Autodesk Inventor part; units mm, degrees
(part 2 of 3)
  line L186 (-35.1562, 49.0328) -> (-35.1562, 44.7064)
  spline S339 degree 2 poles (-35.1562, 44.7064) (-35.1562, 44.3627) (-35.4862, 44.3627) knots 0 0 0 1 1 1
  spline S340 degree 2 poles (-35.4862, 44.3627) (-35.7062, 44.3627) (-35.8666, 44.601) knots 0 0 0 1 1 1
  line L187 (-35.8666, 44.601) -> (-38.1443, 48.1025)
  line L188 (-38.1443, 48.1025) -> (-38.1443, 44.7248)
  spline S341 degree 2 poles (-38.1443, 44.7248) (-38.1443, 44.3627) (-38.4926, 44.3627) knots 0 0 0 1 1 1
  spline S342 degree 2 poles (-38.4926, 44.3627) (-38.8409, 44.3627) (-38.8409, 44.7248) knots 0 0 0 1 1 1
  line L189 (-38.8409, 44.7248) -> (-38.8409, 49.042)
  spline S343 degree 2 poles (-43.4515, 49.042) (-43.4515, 49.3949) (-43.1444, 49.3949) knots 0 0 0 1 1 1
  spline S344 degree 2 poles (-43.1444, 49.3949) (-42.9428, 49.3949) (-42.8098, 49.2024) knots 0 0 0 1 1 1
  line L190 (-42.8098, 49.2024) -> (-40.4633, 45.6093)
  line L191 (-40.4633, 45.6093) -> (-40.4633, 49.0328)
  spline S345 degree 2 poles (-40.4633, 49.0328) (-40.4633, 49.3949) (-40.115, 49.3949) knots 0 0 0 1 1 1
  spline S346 degree 2 poles (-40.115, 49.3949) (-39.7667, 49.3949) (-39.7667, 49.0328) knots 0 0 0 1 1 1
  line L192 (-39.7667, 49.0328) -> (-39.7667, 44.7064)
  spline S347 degree 2 poles (-39.7667, 44.7064) (-39.7667, 44.3627) (-40.0967, 44.3627) knots 0 0 0 1 1 1
  spline S348 degree 2 poles (-40.0967, 44.3627) (-40.3167, 44.3627) (-40.4771, 44.601) knots 0 0 0 1 1 1
  line L193 (-40.4771, 44.601) -> (-42.7548, 48.1025)
  line L194 (-42.7548, 48.1025) -> (-42.7548, 44.7248)
  spline S349 degree 2 poles (-42.7548, 44.7248) (-42.7548, 44.3627) (-43.1032, 44.3627) knots 0 0 0 1 1 1
  spline S350 degree 2 poles (-43.1032, 44.3627) (-43.4515, 44.3627) (-43.4515, 44.7248) knots 0 0 0 1 1 1
  line L195 (-43.4515, 44.7248) -> (-43.4515, 49.042)
  spline S351 degree 2 poles (-56.2885, 49.042) (-56.2885, 49.404) (-55.9402, 49.404) knots 0 0 0 1 1 1
  spline S352 degree 2 poles (-55.9402, 49.404) (-55.5873, 49.404) (-55.5873, 49.042) knots 0 0 0 1 1 1
  line L196 (-55.5873, 49.042) -> (-55.5873, 44.436)
  line L197 (-55.5873, 44.436) -> (-54.1986, 46.6313)
  spline S353 degree 2 poles (-54.1986, 46.6313) (-54.0382, 46.865) (-53.8091, 46.865) knots 0 0 0 1 1 1
  spline S354 degree 2 poles (-53.8091, 46.865) (-53.5891, 46.865) (-53.4745, 46.6955) knots 0 0 0 1 1 1
  line L198 (-53.4745, 46.6955) -> (-52.0584, 44.4177)
  line L199 (-52.0584, 44.4177) -> (-52.0584, 49.042)
  spline S355 degree 2 poles (-52.0584, 49.042) (-52.0584, 49.404) (-51.7009, 49.404) knots 0 0 0 1 1 1
  spline S356 degree 2 poles (-51.7009, 49.404) (-51.348, 49.404) (-51.348, 49.042) knots 0 0 0 1 1 1
  line L200 (-51.348, 49.042) -> (-51.348, 43.7211)
  spline S357 degree 2 poles (-51.348, 43.7211) (-51.348, 43.3407) (-51.7284, 43.3407) knots 0 0 0 1 1 1
  spline S358 degree 2 poles (-51.7284, 43.3407) (-52.0217, 43.3407) (-52.2142, 43.6111) knots 0 0 0 1 1 1
  line L201 (-52.2142, 43.6111) -> (-53.8183, 45.9805)
  line L202 (-53.8183, 45.9805) -> (-55.459, 43.5836)
  spline S359 degree 2 poles (-55.459, 43.5836) (-55.6469, 43.304) (-55.9127, 43.304) knots 0 0 0 1 1 1
  spline S360 degree 2 poles (-55.9127, 43.304) (-56.2885, 43.304) (-56.2885, 43.7165) knots 0 0 0 1 1 1
  line L203 (-56.2885, 43.7165) -> (-56.2885, 49.042)
  spline S361 degree 2 poles (-61.2748, 46.8925) (-61.2748, 47.8641) (-60.7844, 48.5928) knots 0 0 0 1 1 1
  spline S362 degree 2 poles (-60.7844, 48.5928) (-60.2437, 49.3949) (-59.3958, 49.3949) knots 0 0 0 1 1 1
  spline S363 degree 2 poles (-59.3958, 49.3949) (-58.5479, 49.3949) (-58.0071, 48.5837) knots 0 0 0 1 1 1
  spline S364 degree 2 poles (-58.0071, 48.5837) (-57.5213, 47.855) (-57.5213, 46.8925) knots 0 0 0 1 1 1
  spline S365 degree 2 poles (-57.5213, 46.8925) (-57.5213, 45.9347) (-58.0026, 45.2243) knots 0 0 0 1 1 1
  spline S366 degree 2 poles (-58.0026, 45.2243) (-58.5663, 44.404) (-59.3958, 44.404) knots 0 0 0 1 1 1
  spline S367 degree 2 poles (-59.3958, 44.404) (-60.2803, 44.404) (-60.7524, 45.1693) knots 0 0 0 1 1 1
  spline S368 degree 2 poles (-60.7524, 45.1693) (-61.2748, 45.9209) (-61.2748, 46.8925) knots 0 0 0 1 1 1
  spline S369 degree 2 poles (-60.5782, 46.8925) (-60.5782, 46.1776) (-60.3124, 45.7193) knots 0 0 0 1 1 1
  spline S370 degree 2 poles (-60.3124, 45.7193) (-59.9687, 45.1098) (-59.3958, 45.1098) knots 0 0 0 1 1 1
  spline S371 degree 2 poles (-59.3958, 45.1098) (-58.8596, 45.1098) (-58.5204, 45.678) knots 0 0 0 1 1 1
  spline S372 degree 2 poles (-58.5204, 45.678) (-58.218, 46.1913) (-58.218, 46.8925) knots 0 0 0 1 1 1
  spline S373 degree 2 poles (-58.218, 46.8925) (-58.218, 47.6121) (-58.3738, 48.0795) knots 0 0 0 1 1 1
  spline S374 degree 2 poles (-58.3738, 48.0795) (-58.8412, 48.6891) (-59.3958, 48.6891) knots 0 0 0 1 1 1
  spline S375 degree 2 poles (-59.3958, 48.6891) (-59.9549, 48.6891) (-60.4224, 48.0795) knots 0 0 0 1 1 1
  spline S376 degree 2 poles (-60.4224, 48.0795) (-60.5782, 47.6075) (-60.5782, 46.8925) knots 0 0 0 1 1 1
  spline S377 degree 2 poles (-65.6883, 45.8064) (-65.6883, 46.5626) (-65.2162, 46.9109) knots 0 0 0 1 1 1
  spline S378 degree 2 poles (-65.2162, 46.9109) (-64.8404, 47.2179) (-64.4967, 47.2179) knots 0 0 0 1 1 1
  line L204 (-64.4967, 47.2179) -> (-64.4554, 47.2134)
  line L205 (-64.4554, 47.2134) -> (-65.6195, 48.8312)
  spline S379 degree 2 poles (-65.6195, 48.8312) (-65.6883, 48.9412) (-65.6883, 49.042) knots 0 0 0 1 1 1
  spline S380 degree 2 poles (-65.6883, 49.042) (-65.6883, 49.1886) (-65.4729, 49.404) (-65.3308, 49.404) knots 0 0 0 1 2 2 2
  spline S381 degree 2 poles (-65.3308, 49.404) (-65.1658, 49.404) (-65.1246, 49.294) knots 0 0 0 1 1 1
  line L206 (-65.1246, 49.294) -> (-63.6763, 47.2179)
  line L207 (-63.6763, 47.2179) -> (-62.8285, 47.2179)
  line L208 (-62.8285, 47.2179) -> (-62.8285, 49.042)
  spline S382 degree 2 poles (-62.8285, 49.042) (-62.8285, 49.404) (-62.4802, 49.404) knots 0 0 0 1 1 1
  spline S383 degree 2 poles (-62.4802, 49.404) (-62.1319, 49.404) (-62.1319, 49.042) knots 0 0 0 1 1 1
  line L209 (-62.1319, 49.042) -> (-62.1319, 44.3902)
  line L210 (-62.1319, 44.3902) -> (-64.24, 44.3902)
  spline S384 degree 2 poles (-64.24, 44.3902) (-64.8404, 44.3902) (-65.2437, 44.7477) knots 0 0 0 1 1 1
  spline S385 degree 2 poles (-65.2437, 44.7477) (-65.6883, 45.1464) (-65.6883, 45.8064) knots 0 0 0 1 1 1
  spline S386 degree 2 poles (-64.9917, 45.8064) (-64.9917, 45.4626) (-64.5563, 45.096) (-64.24, 45.096) knots 0 0 0 1 2 2 2
  line L211 (-64.24, 45.096) -> (-62.8285, 45.096)
  line L212 (-62.8285, 45.096) -> (-62.8285, 46.5122)
  line L213 (-62.8285, 46.5122) -> (-64.4967, 46.5122)
  spline S387 degree 2 poles (-64.4967, 46.5122) (-64.625, 46.5122) (-64.7854, 46.3655) knots 0 0 0 1 1 1
  spline S388 degree 2 poles (-64.7854, 46.3655) (-64.9917, 46.173) (-64.9917, 45.8064) knots 0 0 0 1 1 1
  spline S389 degree 2 poles (-70.5371, 48.9182) (-70.56, 48.987) (-70.56, 49.0511) knots 0 0 0 1 1 1
  spline S390 degree 2 poles (-70.56, 49.0511) (-70.56, 49.2024) (-70.3309, 49.3949) (-70.1934, 49.3949) knots 0 0 0 1 2 2 2
  spline S391 degree 2 poles (-70.1934, 49.3949) (-69.9597, 49.3949) (-69.8817, 49.1749) knots 0 0 0 1 1 1
  line L214 (-69.8817, 49.1749) -> (-69.5976, 48.4829)
  line L215 (-69.5976, 48.4829) -> (-67.3611, 48.4829)
  line L216 (-67.3611, 48.4829) -> (-67.0999, 49.1703)
  spline S392 degree 2 poles (-67.0999, 49.1703) (-67.0036, 49.3949) (-66.7699, 49.3949) knots 0 0 0 1 1 1
  spline S393 degree 2 poles (-66.7699, 49.3949) (-66.417, 49.3949) (-66.417, 49.0557) knots 0 0 0 1 1 1
  spline S394 degree 2 poles (-66.417, 49.0557) (-66.417, 48.9916) (-66.4353, 48.9366) knots 0 0 0 1 1 1
  line L217 (-66.4353, 48.9366) -> (-68.0944, 44.5598)
  spline S395 degree 2 poles (-68.0944, 44.5598) (-68.2364, 44.3444) (-68.4473, 44.3444) knots 0 0 0 1 1 1
  spline S396 degree 2 poles (-68.4473, 44.3444) (-68.6581, 44.3444) (-68.8047, 44.5552) knots 0 0 0 1 1 1
  line L218 (-68.8047, 44.5552) -> (-70.5371, 48.9182)
  line L219 (-69.3639, 47.7862) -> (-68.4564, 45.3985)
  line L220 (-68.4564, 45.3985) -> (-67.5765, 47.7862)
  line L221 (-67.5765, 47.7862) -> (-69.3639, 47.7862)
  spline S397 degree 2 poles (-75.0789, 49.042) (-75.0789, 49.3949) (-74.7718, 49.3949) knots 0 0 0 1 1 1
  spline S398 degree 2 poles (-74.7718, 49.3949) (-74.5702, 49.3949) (-74.4373, 49.2024) knots 0 0 0 1 1 1
  line L222 (-74.4373, 49.2024) -> (-72.0908, 45.6093)
  line L223 (-72.0908, 45.6093) -> (-72.0908, 49.0328)
  spline S399 degree 2 poles (-72.0908, 49.0328) (-72.0908, 49.3949) (-71.7425, 49.3949) knots 0 0 0 1 1 1
  spline S400 degree 2 poles (-71.7425, 49.3949) (-71.3941, 49.3949) (-71.3941, 49.0328) knots 0 0 0 1 1 1
  line L224 (-71.3941, 49.0328) -> (-71.3941, 44.7064)
  spline S401 degree 2 poles (-71.3941, 44.7064) (-71.3941, 44.3627) (-71.7241, 44.3627) knots 0 0 0 1 1 1
  spline S402 degree 2 poles (-71.7241, 44.3627) (-71.9441, 44.3627) (-72.1045, 44.601) knots 0 0 0 1 1 1
  line L225 (-72.1045, 44.601) -> (-74.3823, 48.1025)
  line L226 (-74.3823, 48.1025) -> (-74.3823, 44.7248)
  spline S403 degree 2 poles (-74.3823, 44.7248) (-74.3823, 44.3627) (-74.7306, 44.3627) knots 0 0 0 1 1 1
  spline S404 degree 2 poles (-74.7306, 44.3627) (-75.0789, 44.3627) (-75.0789, 44.7248) knots 0 0 0 1 1 1
  line L227 (-75.0789, 44.7248) -> (-75.0789, 49.042)
  spline S405 degree 2 poles (-79.639, 46.7367) (-79.639, 47.9329) (-79.0982, 48.5791) knots 0 0 0 1 1 1
  spline S406 degree 2 poles (-79.0982, 48.5791) (-78.7636, 49.0695) (-77.9845, 49.2207) knots 0 0 0 1 1 1
  spline S407 degree 2 poles (-77.9845, 49.2207) (-77.43, 49.3261) (-76.1834, 49.3261) knots 0 0 0 1 1 1
  line L228 (-76.1834, 49.3261) -> (-76.1834, 44.3902)
  spline S408 degree 2 poles (-76.1834, 44.3902) (-77.9937, 44.3902) (-78.6216, 44.6927) knots 0 0 0 1 1 1
  spline S409 degree 2 poles (-78.6216, 44.6927) (-79.639, 45.1831) (-79.639, 46.7367) knots 0 0 0 1 1 1
  spline S410 degree 2 poles (-78.9515, 46.7367) (-78.9515, 45.6551) (-78.2916, 45.3114) knots 0 0 0 1 1 1
  spline S411 degree 2 poles (-78.2916, 45.3114) (-77.8654, 45.0868) (-76.8846, 45.0868) knots 0 0 0 1 1 1
  line L229 (-76.8846, 45.0868) -> (-76.8846, 48.6203)
  spline S412 degree 2 poles (-76.8846, 48.6203) (-77.8608, 48.6203) (-78.3099, 48.3545) knots 0 0 0 1 1 1
  spline S413 degree 2 poles (-78.3099, 48.3545) (-78.9515, 47.9696) (-78.9515, 46.7367) knots 0 0 0 1 1 1
  line L230 (-14.1751, 52.786) -> (-11.187, 52.786)
  line L231 (-11.187, 52.786) -> (-11.187, 54.4268)
  line L232 (-11.187, 54.4268) -> (-13.4785, 54.4268)
  spline S414 degree 2 poles (-13.4785, 54.4268) (-13.8452, 54.4268) (-13.8452, 54.7797) knots 0 0 0 1 1 1
  spline S415 degree 2 poles (-13.8452, 54.7797) (-13.8452, 55.1325) (-13.4785, 55.1325) knots 0 0 0 1 1 1
  line L233 (-13.4785, 55.1325) -> (-11.187, 55.1325)
  line L234 (-11.187, 55.1325) -> (-11.187, 57.7632)
  spline S416 degree 2 poles (-11.187, 57.7632) (-11.187, 58.1253) (-10.8387, 58.1253) knots 0 0 0 1 1 1
  spline S417 degree 2 poles (-10.8387, 58.1253) (-10.4858, 58.1253) (-10.4858, 57.7632) knots 0 0 0 1 1 1
  line L235 (-10.4858, 57.7632) -> (-10.4858, 52.0803)
  line L236 (-10.4858, 52.0803) -> (-14.1751, 52.0803)
  spline S418 degree 2 poles (-14.1751, 52.0803) (-14.5326, 52.0803) (-14.5326, 52.4331) knots 0 0 0 1 1 1
  spline S419 degree 2 poles (-14.5326, 52.4331) (-14.5326, 52.786) (-14.1751, 52.786) knots 0 0 0 1 1 1
  line L237 (-18.6115, 58.0748) -> (-15.6279, 58.0748)
  line L238 (-15.6279, 58.0748) -> (-15.6279, 53.1389)
  line L239 (-15.6279, 53.1389) -> (-18.6115, 53.1389)
  spline S420 degree 2 poles (-18.6115, 53.1389) (-18.969, 53.1389) (-18.969, 53.4827) knots 0 0 0 1 1 1
  spline S421 degree 2 poles (-18.969, 53.4827) (-18.969, 53.8356) (-18.6115, 53.8356) knots 0 0 0 1 1 1
  line L240 (-18.6115, 53.8356) -> (-16.3246, 53.8356)
  line L241 (-16.3246, 53.8356) -> (-16.3246, 54.9951)
  line L242 (-16.3246, 54.9951) -> (-18.474, 54.9951)
  spline S422 degree 2 poles (-18.474, 54.9951) (-18.8223, 54.9951) (-18.8223, 55.3479) knots 0 0 0 1 1 1
  spline S423 degree 2 poles (-18.8223, 55.3479) (-18.8223, 55.7008) (-18.474, 55.7008) knots 0 0 0 1 1 1
  line L243 (-18.474, 55.7008) -> (-16.3246, 55.7008)
  line L244 (-16.3246, 55.7008) -> (-16.3246, 57.3691)
  line L245 (-16.3246, 57.3691) -> (-18.6115, 57.3691)
  spline S424 degree 2 poles (-18.6115, 57.3691) (-18.969, 57.3691) (-18.969, 57.722) knots 0 0 0 1 1 1
  spline S425 degree 2 poles (-18.969, 57.722) (-18.969, 58.0748) (-18.6115, 58.0748) knots 0 0 0 1 1 1
  line L246 (-22.9379, 58.0748) -> (-19.9543, 58.0748)
  line L247 (-19.9543, 58.0748) -> (-19.9543, 53.4918)
  spline S426 degree 2 poles (-19.9543, 53.4918) (-19.9543, 53.1298) (-20.3026, 53.1298) knots 0 0 0 1 1 1
  spline S427 degree 2 poles (-20.3026, 53.1298) (-20.6509, 53.1298) (-20.6509, 53.4918) knots 0 0 0 1 1 1
  line L248 (-20.6509, 53.4918) -> (-20.6509, 57.3691)
  line L249 (-20.6509, 57.3691) -> (-22.9379, 57.3691)
  spline S428 degree 2 poles (-22.9379, 57.3691) (-23.2953, 57.3691) (-23.2953, 57.722) knots 0 0 0 1 1 1
  spline S429 degree 2 poles (-23.2953, 57.722) (-23.2953, 58.0748) (-22.9379, 58.0748) knots 0 0 0 1 1 1
  spline S430 degree 2 poles (-24.9177, 57.7815) (-24.9177, 58.1436) (-24.5603, 58.1436) knots 0 0 0 1 1 1
  spline S431 degree 2 poles (-24.5603, 58.1436) (-24.2074, 58.1436) (-24.2074, 57.7815) knots 0 0 0 1 1 1
  line L250 (-24.2074, 57.7815) -> (-24.2074, 53.4918)
  spline S432 degree 2 poles (-24.2074, 53.4918) (-24.2074, 53.1298) (-24.5603, 53.1298) knots 0 0 0 1 1 1
  spline S433 degree 2 poles (-24.5603, 53.1298) (-24.9177, 53.1298) (-24.9177, 53.4918) knots 0 0 0 1 1 1
  line L251 (-24.9177, 53.4918) -> (-24.9177, 57.7815)
  spline S434 degree 2 poles (-29.4595, 54.4955) (-29.4595, 55.0775) (-29.1524, 55.4304) knots 0 0 0 1 1 1
  spline S435 degree 2 poles (-29.1524, 55.4304) (-28.827, 55.8108) (-28.2404, 55.8108) knots 0 0 0 1 1 1
  line L252 (-28.2404, 55.8108) -> (-26.9068, 55.8108)
  line L253 (-26.9068, 55.8108) -> (-26.9068, 57.7999)
  spline S436 degree 2 poles (-26.9068, 57.7999) (-26.9068, 58.1619) (-26.5585, 58.1619) knots 0 0 0 1 1 1
  spline S437 degree 2 poles (-26.5585, 58.1619) (-26.2101, 58.1619) (-26.2101, 57.7999) knots 0 0 0 1 1 1
  line L254 (-26.2101, 57.7999) -> (-26.2101, 53.1389)
  line L255 (-26.2101, 53.1389) -> (-28.1304, 53.1389)
  spline S438 degree 2 poles (-28.1304, 53.1389) (-29.4595, 53.1389) (-29.4595, 54.4955) knots 0 0 0 1 1 1
  spline S439 degree 2 poles (-28.7629, 54.4955) (-28.7629, 53.8447) (-28.1304, 53.8447) knots 0 0 0 1 1 1
  line L256 (-28.1304, 53.8447) -> (-26.9068, 53.8447)
  line L257 (-26.9068, 53.8447) -> (-26.9068, 55.105)
  line L258 (-26.9068, 55.105) -> (-28.2404, 55.105)
  spline S440 degree 2 poles (-28.2404, 55.105) (-28.7629, 55.105) (-28.7629, 54.4955) knots 0 0 0 1 1 1
  line L259 (-33.1855, 58.0748) -> (-30.202, 58.0748)
  line L260 (-30.202, 58.0748) -> (-30.202, 53.1389)
  line L261 (-30.202, 53.1389) -> (-33.1855, 53.1389)
  spline S441 degree 2 poles (-33.1855, 53.1389) (-33.543, 53.1389) (-33.543, 53.4827) knots 0 0 0 1 1 1
  spline S442 degree 2 poles (-33.543, 53.4827) (-33.543, 53.8356) (-33.1855, 53.8356) knots 0 0 0 1 1 1
  line L262 (-33.1855, 53.8356) -> (-30.8986, 53.8356)
  line L263 (-30.8986, 53.8356) -> (-30.8986, 54.9951)
  line L264 (-30.8986, 54.9951) -> (-33.048, 54.9951)
  spline S443 degree 2 poles (-33.048, 54.9951) (-33.3963, 54.9951) (-33.3963, 55.3479) knots 0 0 0 1 1 1
  spline S444 degree 2 poles (-33.3963, 55.3479) (-33.3963, 55.7008) (-33.048, 55.7008) knots 0 0 0 1 1 1
  line L265 (-33.048, 55.7008) -> (-30.8986, 55.7008)
  line L266 (-30.8986, 55.7008) -> (-30.8986, 57.3691)
  line L267 (-30.8986, 57.3691) -> (-33.1855, 57.3691)
  spline S445 degree 2 poles (-33.1855, 57.3691) (-33.543, 57.3691) (-33.543, 57.722) knots 0 0 0 1 1 1
  spline S446 degree 2 poles (-33.543, 57.722) (-33.543, 58.0748) (-33.1855, 58.0748) knots 0 0 0 1 1 1
  spline S447 degree 2 poles (-42.2553, 53.8172) (-42.2553, 54.7292) (-41.6503, 55.1875) knots 0 0 0 1 1 1
  spline S448 degree 2 poles (-41.6503, 55.1875) (-41.2425, 55.4946) (-40.8391, 55.4946) knots 0 0 0 1 1 1
  line L268 (-40.8391, 55.4946) -> (-40.6283, 55.4946)
  line L269 (-40.6283, 55.4946) -> (-42.1774, 57.5661)
  spline S449 degree 2 poles (-42.1774, 57.5661) (-42.2553, 57.6807) (-42.2553, 57.7907) knots 0 0 0 1 1 1
  spline S450 degree 2 poles (-42.2553, 57.7907) (-42.2553, 57.9282) (-42.0399, 58.1436) (-41.8978, 58.1436) knots 0 0 0 1 2 2 2
  spline S451 degree 2 poles (-41.8978, 58.1436) (-41.7237, 58.1436) (-41.6503, 58.0336) knots 0 0 0 1 1 1
  line L270 (-41.6503, 58.0336) -> (-39.8309, 55.4946)
  line L271 (-39.8309, 55.4946) -> (-38.6255, 55.4946)
  line L272 (-38.6255, 55.4946) -> (-38.6255, 57.7815)
  spline S452 degree 2 poles (-38.6255, 57.7815) (-38.6255, 58.1436) (-38.2681, 58.1436) knots 0 0 0 1 1 1
  spline S453 degree 2 poles (-38.2681, 58.1436) (-37.9152, 58.1436) (-37.9152, 57.7815) knots 0 0 0 1 1 1
  line L273 (-37.9152, 57.7815) -> (-37.9152, 52.0803)
  line L274 (-37.9152, 52.0803) -> (-40.5137, 52.0803)
  spline S454 degree 2 poles (-40.5137, 52.0803) (-41.2195, 52.0803) (-41.7191, 52.534) knots 0 0 0 1 1 1
  spline S455 degree 2 poles (-41.7191, 52.534) (-42.2553, 53.0244) (-42.2553, 53.8172) knots 0 0 0 1 1 1
  spline S456 degree 2 poles (-41.5541, 53.8172) (-41.5541, 53.3406) (-41.2425, 53.0519) knots 0 0 0 1 1 1
  spline S457 degree 2 poles (-41.2425, 53.0519) (-40.9446, 52.786) (-40.5137, 52.786) knots 0 0 0 1 1 1
  line L275 (-40.5137, 52.786) -> (-38.6255, 52.786)
  line L276 (-38.6255, 52.786) -> (-38.6255, 54.7797)
  line L277 (-38.6255, 54.7797) -> (-40.8391, 54.7797)
  spline S458 degree 2 poles (-40.8391, 54.7797) (-41.0316, 54.7797) (-41.247, 54.5963) knots 0 0 0 1 1 1
  spline S459 degree 2 poles (-41.247, 54.5963) (-41.5541, 54.3351) (-41.5541, 53.8172) knots 0 0 0 1 1 1
  spline S460 degree 2 poles (-47.3562, 57.667) (-47.3791, 57.7357) (-47.3791, 57.7999) knots 0 0 0 1 1 1
  spline S461 degree 2 poles (-47.3791, 57.7999) (-47.3791, 57.9511) (-47.15, 58.1436) (-47.0125, 58.1436) knots 0 0 0 1 2 2 2
  spline S462 degree 2 poles (-47.0125, 58.1436) (-46.7787, 58.1436) (-46.7008, 57.9236) knots 0 0 0 1 1 1
  line L278 (-46.7008, 57.9236) -> (-46.4167, 57.2316)
  line L279 (-46.4167, 57.2316) -> (-44.1802, 57.2316)
  line L280 (-44.1802, 57.2316) -> (-43.9189, 57.919)
  spline S463 degree 2 poles (-43.9189, 57.919) (-43.8227, 58.1436) (-43.589, 58.1436) knots 0 0 0 1 1 1
  spline S464 degree 2 poles (-43.589, 58.1436) (-43.2361, 58.1436) (-43.2361, 57.8044) knots 0 0 0 1 1 1
  spline S465 degree 2 poles (-43.2361, 57.8044) (-43.2361, 57.7403) (-43.2544, 57.6853) knots 0 0 0 1 1 1
  line L281 (-43.2544, 57.6853) -> (-44.9134, 53.3085)
  spline S466 degree 2 poles (-44.9134, 53.3085) (-45.0555, 53.0931) (-45.2663, 53.0931) knots 0 0 0 1 1 1
  spline S467 degree 2 poles (-45.2663, 53.0931) (-45.4772, 53.0931) (-45.6238, 53.3039) knots 0 0 0 1 1 1
  line L282 (-45.6238, 53.3039) -> (-47.3562, 57.667)
  line L283 (-46.1829, 56.535) -> (-45.2755, 54.1472)
  line L284 (-45.2755, 54.1472) -> (-44.3956, 56.535)
  line L285 (-44.3956, 56.535) -> (-46.1829, 56.535)
  spline S468 degree 2 poles (-52.2967, 57.7815) (-52.2967, 58.1436) (-51.953, 58.1436) knots 0 0 0 1 1 1
  spline S469 degree 2 poles (-51.953, 58.1436) (-51.6092, 58.1436) (-51.6092, 57.7815) knots 0 0 0 1 1 1
  line L286 (-51.6092, 57.7815) -> (-51.6092, 54.2572)
  line L287 (-51.6092, 54.2572) -> (-50.6193, 55.8979)
  spline S470 degree 2 poles (-50.6193, 55.8979) (-50.4818, 56.0996) (-50.2527, 56.0996) knots 0 0 0 1 1 1
  spline S471 degree 2 poles (-50.2527, 56.0996) (-50.0235, 56.0996) (-49.8952, 55.9025) knots 0 0 0 1 1 1
  line L288 (-49.8952, 55.9025) -> (-48.9144, 54.2389)
  line L289 (-48.9144, 54.2389) -> (-48.9144, 57.7815)
  spline S472 degree 2 poles (-48.9144, 57.7815) (-48.9144, 58.1436) (-48.5661, 58.1436) knots 0 0 0 1 1 1
  spline S473 degree 2 poles (-48.5661, 58.1436) (-48.2132, 58.1436) (-48.2132, 57.7815) knots 0 0 0 1 1 1
  line L290 (-48.2132, 57.7815) -> (-48.2132, 53.5285)
  spline S474 degree 2 poles (-48.2132, 53.5285) (-48.2132, 53.1481) (-48.5844, 53.1481) knots 0 0 0 1 1 1
  spline S475 degree 2 poles (-48.5844, 53.1481) (-48.8548, 53.1481) (-49.029, 53.4002) knots 0 0 0 1 1 1
  line L291 (-49.029, 53.4002) -> (-50.2527, 55.238)
  line L292 (-50.2527, 55.238) -> (-51.4855, 53.4093)
  spline S476 degree 2 poles (-51.4855, 53.4093) (-51.6872, 53.1206) (-51.9392, 53.1206) knots 0 0 0 1 1 1
  spline S477 degree 2 poles (-51.9392, 53.1206) (-52.2967, 53.1206) (-52.2967, 53.5239) knots 0 0 0 1 1 1
  line L293 (-52.2967, 53.5239) -> (-52.2967, 57.7815)
  spline S478 degree 2 poles (-54.4415, 57.7815) (-54.4415, 58.1436) (-54.0841, 58.1436) knots 0 0 0 1 1 1
  spline S479 degree 2 poles (-54.0841, 58.1436) (-53.7312, 58.1436) (-53.7312, 57.7815) knots 0 0 0 1 1 1
  line L294 (-53.7312, 57.7815) -> (-53.7312, 53.4918)
  spline S480 degree 2 poles (-53.7312, 53.4918) (-53.7312, 53.1298) (-54.0841, 53.1298) knots 0 0 0 1 1 1
  spline S481 degree 2 poles (-54.0841, 53.1298) (-54.4415, 53.1298) (-54.4415, 53.4918) knots 0 0 0 1 1 1
  line L295 (-54.4415, 53.4918) -> (-54.4415, 57.7815)
  spline S482 degree 2 poles (-59.2904, 54.5551) (-59.2904, 55.3113) (-58.8183, 55.6596) knots 0 0 0 1 1 1
  spline S483 degree 2 poles (-58.8183, 55.6596) (-58.4425, 55.9667) (-58.0988, 55.9667) knots 0 0 0 1 1 1
  line L296 (-58.0988, 55.9667) -> (-58.0576, 55.9621)
  line L297 (-58.0576, 55.9621) -> (-59.2216, 57.5799)
  spline S484 degree 2 poles (-59.2216, 57.5799) (-59.2904, 57.6899) (-59.2904, 57.7907) knots 0 0 0 1 1 1
  spline S485 degree 2 poles (-59.2904, 57.7907) (-59.2904, 57.9374) (-59.075, 58.1528) (-58.9329, 58.1528) knots 0 0 0 1 2 2 2
  spline S486 degree 2 poles (-58.9329, 58.1528) (-58.7679, 58.1528) (-58.7267, 58.0428) knots 0 0 0 1 1 1
  line L298 (-58.7267, 58.0428) -> (-57.2784, 55.9667)
  line L299 (-57.2784, 55.9667) -> (-56.4306, 55.9667)
  line L300 (-56.4306, 55.9667) -> (-56.4306, 57.7907)
  spline S487 degree 2 poles (-56.4306, 57.7907) (-56.4306, 58.1528) (-56.0823, 58.1528) knots 0 0 0 1 1 1
  spline S488 degree 2 poles (-56.0823, 58.1528) (-55.734, 58.1528) (-55.734, 57.7907) knots 0 0 0 1 1 1
  line L301 (-55.734, 57.7907) -> (-55.734, 53.1389)
  line L302 (-55.734, 53.1389) -> (-57.8421, 53.1389)
  spline S489 degree 2 poles (-57.8421, 53.1389) (-58.4425, 53.1389) (-58.8458, 53.4964) knots 0 0 0 1 1 1
  spline S490 degree 2 poles (-58.8458, 53.4964) (-59.2904, 53.8951) (-59.2904, 54.5551) knots 0 0 0 1 1 1
  spline S491 degree 2 poles (-58.5938, 54.5551) (-58.5938, 54.2114) (-58.1584, 53.8447) (-57.8421, 53.8447) knots 0 0 0 1 2 2 2
  line L303 (-57.8421, 53.8447) -> (-56.4306, 53.8447)
  line L304 (-56.4306, 53.8447) -> (-56.4306, 55.2609)
  line L305 (-56.4306, 55.2609) -> (-58.0988, 55.2609)
  spline S492 degree 2 poles (-58.0988, 55.2609) (-58.2271, 55.2609) (-58.3875, 55.1142) knots 0 0 0 1 1 1
  spline S493 degree 2 poles (-58.3875, 55.1142) (-58.5938, 54.9217) (-58.5938, 54.5551) knots 0 0 0 1 1 1
  line L306 (-63.053, 58.0748) -> (-60.0695, 58.0748)
  line L307 (-60.0695, 58.0748) -> (-60.0695, 53.1389)
  line L308 (-60.0695, 53.1389) -> (-63.053, 53.1389)
  spline S494 degree 2 poles (-63.053, 53.1389) (-63.4105, 53.1389) (-63.4105, 53.4827) knots 0 0 0 1 1 1
  spline S495 degree 2 poles (-63.4105, 53.4827) (-63.4105, 53.8356) (-63.053, 53.8356) knots 0 0 0 1 1 1
  line L309 (-63.053, 53.8356) -> (-60.7661, 53.8356)
  line L310 (-60.7661, 53.8356) -> (-60.7661, 54.9951)
  line L311 (-60.7661, 54.9951) -> (-62.9156, 54.9951)
  spline S496 degree 2 poles (-62.9156, 54.9951) (-63.2639, 54.9951) (-63.2639, 55.3479) knots 0 0 0 1 1 1
  spline S497 degree 2 poles (-63.2639, 55.3479) (-63.2639, 55.7008) (-62.9156, 55.7008) knots 0 0 0 1 1 1
  line L312 (-62.9156, 55.7008) -> (-60.7661, 55.7008)
  line L313 (-60.7661, 55.7008) -> (-60.7661, 57.3691)
  line L314 (-60.7661, 57.3691) -> (-63.053, 57.3691)
  spline S498 degree 2 poles (-63.053, 57.3691) (-63.4105, 57.3691) (-63.4105, 57.722) knots 0 0 0 1 1 1
  spline S499 degree 2 poles (-63.4105, 57.722) (-63.4105, 58.0748) (-63.053, 58.0748) knots 0 0 0 1 1 1
  line L315 (-67.5673, 53.611) -> (-65.1475, 57.3691)
  line L316 (-65.1475, 57.3691) -> (-67.3198, 57.3691)
  spline S500 degree 2 poles (-67.3198, 57.3691) (-67.6773, 57.3691) (-67.6773, 57.722) knots 0 0 0 1 1 1
  spline S501 degree 2 poles (-67.6773, 57.722) (-67.6773, 58.0748) (-67.3198, 58.0748) knots 0 0 0 1 1 1
  line L317 (-67.3198, 58.0748) -> (-64.4738, 58.0748)
  spline S502 degree 2 poles (-64.4738, 58.0748) (-64.2217, 58.0748) (-64.2217, 57.7999) knots 0 0 0 1 1 1
  spline S503 degree 2 poles (-64.2217, 57.7999) (-64.2217, 57.644) (-64.2813, 57.6624) knots 0 0 0 1 1 1
  line L318 (-64.2813, 57.6624) -> (-66.6874, 53.8356)
  line L319 (-66.6874, 53.8356) -> (-64.5929, 53.8356)
  spline S504 degree 2 poles (-64.5929, 53.8356) (-64.24, 53.8356) (-64.24, 53.4827) knots 0 0 0 1 1 1
  spline S505 degree 2 poles (-64.24, 53.4827) (-64.24, 53.1389) (-64.5929, 53.1389) knots 0 0 0 1 1 1
  line L320 (-64.5929, 53.1389) -> (-67.3794, 53.1389)
  spline S506 degree 2 poles (-67.3794, 53.1389) (-67.6269, 53.1389) (-67.6269, 53.3635) knots 0 0 0 1 1 1
  spline S507 degree 2 poles (-67.6269, 53.3635) (-67.6269, 53.4368) (-67.5673, 53.611) knots 0 0 0 1 1 1
  spline S508 degree 2 poles (-14.4547, 65.137) (-14.4547, 66.8144) (-12.5344, 66.8144) knots 0 0 0 1 1 1
  line L321 (-12.5344, 66.8144) -> (-10.4766, 66.8144)
  line L322 (-10.4766, 66.8144) -> (-10.4766, 60.8106)
  line L323 (-10.4766, 60.8106) -> (-12.3786, 60.8106)
  spline S509 degree 2 poles (-12.3786, 60.8106) (-13.2723, 60.8106) (-14.2989, 61.7318) (-14.2989, 62.4789) knots 0 0 0 1 2 2 2
  spline S510 degree 2 poles (-14.2989, 62.4789) (-14.2989, 63.5055) (-13.5702, 63.7667) knots 0 0 0 1 1 1
  spline S511 degree 2 poles (-13.5702, 63.7667) (-14.4547, 64.0004) (-14.4547, 65.137) knots 0 0 0 1 1 1
  spline S512 degree 2 poles (-13.7535, 65.1187) (-13.7535, 64.1562) (-12.4886, 64.1562) knots 0 0 0 1 1 1
  line L324 (-12.4886, 64.1562) -> (-11.1778, 64.1562)
  line L325 (-11.1778, 64.1562) -> (-11.1778, 66.1086)
  line L326 (-11.1778, 66.1086) -> (-12.5344, 66.1086)
  spline S513 degree 2 poles (-12.5344, 66.1086) (-13.7535, 66.1086) (-13.7535, 65.1187) knots 0 0 0 1 1 1
  spline S514 degree 2 poles (-13.5977, 62.4697) (-13.5977, 62.0251) (-12.956, 61.5256) (-12.3786, 61.5256) knots 0 0 0 1 2 2 2
  line L327 (-12.3786, 61.5256) -> (-11.1778, 61.5256)
  line L328 (-11.1778, 61.5256) -> (-11.1778, 63.4413)
  line L329 (-11.1778, 63.4413) -> (-12.3786, 63.4413)
  spline S515 degree 2 poles (-12.3786, 63.4413) (-13.034, 63.4413) (-13.5977, 63.0059) (-13.5977, 62.4697) knots 0 0 0 1 2 2 2
  spline S516 degree 2 poles (-19.7847, 66.4157) (-19.8077, 66.4844) (-19.8077, 66.5486) knots 0 0 0 1 1 1
  spline S517 degree 2 poles (-19.8077, 66.5486) (-19.8077, 66.6998) (-19.5785, 66.8923) (-19.441, 66.8923) knots 0 0 0 1 2 2 2
  spline S518 degree 2 poles (-19.441, 66.8923) (-19.2073, 66.8923) (-19.1294, 66.6723) knots 0 0 0 1 1 1
  line L330 (-19.1294, 66.6723) -> (-18.8452, 65.9803)
  line L331 (-18.8452, 65.9803) -> (-16.6087, 65.9803)
  line L332 (-16.6087, 65.9803) -> (-16.3475, 66.6677)
  spline S519 degree 2 poles (-16.3475, 66.6677) (-16.2512, 66.8923) (-16.0175, 66.8923) knots 0 0 0 1 1 1
  spline S520 degree 2 poles (-16.0175, 66.8923) (-15.6646, 66.8923) (-15.6646, 66.5532) knots 0 0 0 1 1 1
  spline S521 degree 2 poles (-15.6646, 66.5532) (-15.6646, 66.489) (-15.6829, 66.434) knots 0 0 0 1 1 1
  line L333 (-15.6829, 66.434) -> (-17.342, 62.0572)
  spline S522 degree 2 poles (-17.342, 62.0572) (-17.4841, 61.8418) (-17.6949, 61.8418) knots 0 0 0 1 1 1
  spline S523 degree 2 poles (-17.6949, 61.8418) (-17.9057, 61.8418) (-18.0524, 62.0526) knots 0 0 0 1 1 1
  line L334 (-18.0524, 62.0526) -> (-19.7847, 66.4157)
  line L335 (-18.6115, 65.2837) -> (-17.7041, 62.8959)
  line L336 (-17.7041, 62.8959) -> (-16.8241, 65.2837)
  line L337 (-16.8241, 65.2837) -> (-18.6115, 65.2837)
  spline S524 degree 2 poles (-24.024, 63.2442) (-24.024, 63.8263) (-23.717, 64.1792) knots 0 0 0 1 1 1
  spline S525 degree 2 poles (-23.717, 64.1792) (-23.3916, 64.5595) (-22.805, 64.5595) knots 0 0 0 1 1 1
  line L338 (-22.805, 64.5595) -> (-21.4713, 64.5595)
  line L339 (-21.4713, 64.5595) -> (-21.4713, 66.5486)
  spline S526 degree 2 poles (-21.4713, 66.5486) (-21.4713, 66.9106) (-21.123, 66.9106) knots 0 0 0 1 1 1
  spline S527 degree 2 poles (-21.123, 66.9106) (-20.7747, 66.9106) (-20.7747, 66.5486) knots 0 0 0 1 1 1
  line L340 (-20.7747, 66.5486) -> (-20.7747, 61.8876)
  line L341 (-20.7747, 61.8876) -> (-22.695, 61.8876)
  spline S528 degree 2 poles (-22.695, 61.8876) (-24.024, 61.8876) (-24.024, 63.2442) knots 0 0 0 1 1 1
  spline S529 degree 2 poles (-23.3274, 63.2442) (-23.3274, 62.5934) (-22.695, 62.5934) knots 0 0 0 1 1 1
  line L342 (-22.695, 62.5934) -> (-21.4713, 62.5934)
  line L343 (-21.4713, 62.5934) -> (-21.4713, 63.8538)
  line L344 (-21.4713, 63.8538) -> (-22.805, 63.8538)
  spline S530 degree 2 poles (-22.805, 63.8538) (-23.3274, 63.8538) (-23.3274, 63.2442) knots 0 0 0 1 1 1
  line L345 (-28.0754, 62.6118) -> (-26.893, 62.6118)
  line L346 (-26.893, 62.6118) -> (-26.893, 66.5394)
  spline S531 degree 2 poles (-26.893, 66.5394) (-26.893, 66.9106) (-26.5355, 66.9106) knots 0 0 0 1 1 1
  spline S532 degree 2 poles (-26.5355, 66.9106) (-26.1735, 66.9106) (-26.1735, 66.5394) knots 0 0 0 1 1 1
  line L347 (-26.1735, 66.5394) -> (-26.1735, 62.6118)
  line L348 (-26.1735, 62.6118) -> (-24.9956, 62.6118)
  spline S533 degree 2 poles (-24.9956, 62.6118) (-24.6336, 62.6118) (-24.6336, 62.2497) knots 0 0 0 1 1 1
  spline S534 degree 2 poles (-24.6336, 62.2497) (-24.6336, 61.8876) (-24.9956, 61.8876) knots 0 0 0 1 1 1
  line L349 (-24.9956, 61.8876) -> (-28.0754, 61.8876)
  spline S535 degree 2 poles (-28.0754, 61.8876) (-28.4421, 61.8876) (-28.4421, 62.2497) knots 0 0 0 1 1 1
  spline S536 degree 2 poles (-28.4421, 62.2497) (-28.4421, 62.6118) (-28.0754, 62.6118) knots 0 0 0 1 1 1
  spline S537 degree 2 poles (-30.2249, 66.5302) (-30.2249, 66.8923) (-29.8674, 66.8923) knots 0 0 0 1 1 1
  spline S538 degree 2 poles (-29.8674, 66.8923) (-29.5145, 66.8923) (-29.5145, 66.5302) knots 0 0 0 1 1 1
  line L350 (-29.5145, 66.5302) -> (-29.5145, 62.2405)
  spline S539 degree 2 poles (-29.5145, 62.2405) (-29.5145, 61.8785) (-29.8674, 61.8785) knots 0 0 0 1 1 1
  spline S540 degree 2 poles (-29.8674, 61.8785) (-30.2249, 61.8785) (-30.2249, 62.2405) knots 0 0 0 1 1 1
  line L351 (-30.2249, 62.2405) -> (-30.2249, 66.5302)
  spline S541 degree 2 poles (-34.7621, 65.4807) (-34.7621, 66.9198) (-32.9609, 66.9198) knots 0 0 0 1 1 1
  spline S542 degree 2 poles (-32.9609, 66.9198) (-31.9114, 66.9198) (-31.3202, 65.852) knots 0 0 0 1 1 1
  spline S543 degree 2 poles (-31.3202, 65.852) (-31.2744, 65.774) (-31.2744, 65.6778) knots 0 0 0 1 1 1
  spline S544 degree 2 poles (-31.2744, 65.6778) (-31.2744, 65.522) (-31.5035, 65.2928) (-31.6548, 65.2928) knots 0 0 0 1 2 2 2
  spline S545 degree 2 poles (-31.6548, 65.2928) (-31.8335, 65.2928) (-31.916, 65.4716) knots 0 0 0 1 1 1
  spline S546 degree 2 poles (-31.916, 65.4716) (-32.2551, 66.2232) (-32.9609, 66.2232) knots 0 0 0 1 1 1
  spline S547 degree 2 poles (-32.9609, 66.2232) (-34.0609, 66.2232) (-34.0609, 65.4945) knots 0 0 0 1 1 1
  spline S548 degree 2 poles (-34.0609, 65.4945) (-34.0609, 65.1049) (-33.4421, 64.8208) knots 0 0 0 1 1 1
  spline S549 degree 2 poles (-33.4421, 64.8208) (-32.7043, 64.5229) (-32.081, 64.2708) knots 0 0 0 1 1 1
  spline S550 degree 2 poles (-32.081, 64.2708) (-31.3248, 63.84) (-31.3248, 63.1251) knots 0 0 0 1 1 1
  spline S551 degree 2 poles (-31.3248, 63.1251) (-31.3248, 61.8556) (-32.8784, 61.7914) knots 0 0 0 1 1 1
  spline S552 degree 2 poles (-32.8784, 61.7914) (-33.4742, 61.7639) (-34.3954, 62.3139) (-34.5742, 62.8547) knots 0 0 0 1 2 2 2
  spline S553 degree 2 poles (-34.5742, 62.8547) (-34.6017, 62.9142) (-34.6017, 62.9692) knots 0 0 0 1 1 1
  spline S554 degree 2 poles (-34.6017, 62.9692) (-34.6017, 63.2901) (-34.2396, 63.2901) knots 0 0 0 1 1 1
  spline S555 degree 2 poles (-34.2396, 63.2901) (-33.9875, 63.2901) (-33.9096, 63.0517) knots 0 0 0 1 1 1
  spline S556 degree 2 poles (-33.9096, 63.0517) (-33.818, 62.7813) (-33.2542, 62.4697) (-32.9105, 62.488) knots 0 0 0 1 2 2 2
  spline S557 degree 2 poles (-32.9105, 62.488) (-32.0352, 62.5293) (-32.0352, 63.1067) knots 0 0 0 1 1 1
  spline S558 degree 2 poles (-32.0352, 63.1067) (-32.0352, 63.5146) (-32.6447, 63.785) knots 0 0 0 1 1 1
  spline S559 degree 2 poles (-32.6447, 63.785) (-33.3963, 64.1012) (-34.0059, 64.3304) knots 0 0 0 1 1 1
  spline S560 degree 2 poles (-34.0059, 64.3304) (-34.7621, 64.752) (-34.7621, 65.4807) knots 0 0 0 1 1 1
  line L352 (-38.983, 62.6118) -> (-37.8006, 62.6118)
  line L353 (-37.8006, 62.6118) -> (-37.8006, 66.5394)
  spline S561 degree 2 poles (-37.8006, 66.5394) (-37.8006, 66.9106) (-37.4431, 66.9106) knots 0 0 0 1 1 1
  spline S562 degree 2 poles (-37.4431, 66.9106) (-37.0811, 66.9106) (-37.0811, 66.5394) knots 0 0 0 1 1 1
  line L354 (-37.0811, 66.5394) -> (-37.0811, 62.6118)
  line L355 (-37.0811, 62.6118) -> (-35.9032, 62.6118)
  spline S563 degree 2 poles (-35.9032, 62.6118) (-35.5412, 62.6118) (-35.5412, 62.2497) knots 0 0 0 1 1 1
  spline S564 degree 2 poles (-35.5412, 62.2497) (-35.5412, 61.8876) (-35.9032, 61.8876) knots 0 0 0 1 1 1
  line L356 (-35.9032, 61.8876) -> (-38.983, 61.8876)
  spline S565 degree 2 poles (-38.983, 61.8876) (-39.3497, 61.8876) (-39.3497, 62.2497) knots 0 0 0 1 1 1
  spline S566 degree 2 poles (-39.3497, 62.2497) (-39.3497, 62.6118) (-38.983, 62.6118) knots 0 0 0 1 1 1
  line L357 (-43.1444, 66.8236) -> (-40.1609, 66.8236)
  line L358 (-40.1609, 66.8236) -> (-40.1609, 61.8876)
  line L359 (-40.1609, 61.8876) -> (-43.1444, 61.8876)
  spline S567 degree 2 poles (-43.1444, 61.8876) (-43.5019, 61.8876) (-43.5019, 62.2314) knots 0 0 0 1 1 1
  spline S568 degree 2 poles (-43.5019, 62.2314) (-43.5019, 62.5843) (-43.1444, 62.5843) knots 0 0 0 1 1 1
  line L360 (-43.1444, 62.5843) -> (-40.8575, 62.5843)
  line L361 (-40.8575, 62.5843) -> (-40.8575, 63.7438)
  line L362 (-40.8575, 63.7438) -> (-43.0069, 63.7438)
  spline S569 degree 2 poles (-43.0069, 63.7438) (-43.3552, 63.7438) (-43.3552, 64.0967) knots 0 0 0 1 1 1
  spline S570 degree 2 poles (-43.3552, 64.0967) (-43.3552, 64.4496) (-43.0069, 64.4496) knots 0 0 0 1 1 1
  line L363 (-43.0069, 64.4496) -> (-40.8575, 64.4496)
  line L364 (-40.8575, 64.4496) -> (-40.8575, 66.1178)
  line L365 (-40.8575, 66.1178) -> (-43.1444, 66.1178)
  spline S571 degree 2 poles (-43.1444, 66.1178) (-43.5019, 66.1178) (-43.5019, 66.4707) knots 0 0 0 1 1 1
  spline S572 degree 2 poles (-43.5019, 66.4707) (-43.5019, 66.8236) (-43.1444, 66.8236) knots 0 0 0 1 1 1
  line L366 (-51.9576, 61.5531) -> (-50.3902, 61.5531)
  line L367 (-50.3902, 61.5531) -> (-50.3902, 66.6769)
  spline S573 degree 2 poles (-50.3902, 66.6769) (-50.3902, 67.039) (-50.0235, 67.039) knots 0 0 0 1 1 1
  spline S574 degree 2 poles (-50.0235, 67.039) (-49.6615, 67.039) (-49.6615, 66.6769) knots 0 0 0 1 1 1
  line L368 (-49.6615, 66.6769) -> (-49.6615, 61.5531)
  line L369 (-49.6615, 61.5531) -> (-48.0895, 61.5531)
  spline S575 degree 2 poles (-48.0895, 61.5531) (-47.7274, 61.5531) (-47.7274, 61.1819) knots 0 0 0 1 1 1
  spline S576 degree 2 poles (-47.7274, 61.1819) (-47.7274, 60.8198) (-48.0895, 60.8198) knots 0 0 0 1 1 1
  line L370 (-48.0895, 60.8198) -> (-51.9576, 60.8198)
  spline S577 degree 2 poles (-51.9576, 60.8198) (-52.3242, 60.8198) (-52.3242, 61.1819) knots 0 0 0 1 1 1
  spline S578 degree 2 poles (-52.3242, 61.1819) (-52.3242, 61.5531) (-51.9576, 61.5531) knots 0 0 0 1 1 1
  spline S579 degree 2 poles (-57.448, 66.4157) (-57.4709, 66.4844) (-57.4709, 66.5486) knots 0 0 0 1 1 1
  spline S580 degree 2 poles (-57.4709, 66.5486) (-57.4709, 66.6998) (-57.2418, 66.8923) (-57.1043, 66.8923) knots 0 0 0 1 2 2 2
  spline S581 degree 2 poles (-57.1043, 66.8923) (-56.8705, 66.8923) (-56.7926, 66.6723) knots 0 0 0 1 1 1
  line L371 (-56.7926, 66.6723) -> (-56.5085, 65.9803)
  line L372 (-56.5085, 65.9803) -> (-54.272, 65.9803)
  line L373 (-54.272, 65.9803) -> (-54.0107, 66.6677)
  spline S582 degree 2 poles (-54.0107, 66.6677) (-53.9145, 66.8923) (-53.6808, 66.8923) knots 0 0 0 1 1 1
  spline S583 degree 2 poles (-53.6808, 66.8923) (-53.3279, 66.8923) (-53.3279, 66.5532) knots 0 0 0 1 1 1
  spline S584 degree 2 poles (-53.3279, 66.5532) (-53.3279, 66.489) (-53.3462, 66.434) knots 0 0 0 1 1 1
  line L374 (-53.3462, 66.434) -> (-55.0053, 62.0572)
  spline S585 degree 2 poles (-55.0053, 62.0572) (-55.1473, 61.8418) (-55.3582, 61.8418) knots 0 0 0 1 1 1
  spline S586 degree 2 poles (-55.3582, 61.8418) (-55.569, 61.8418) (-55.7156, 62.0526) knots 0 0 0 1 1 1
  line L375 (-55.7156, 62.0526) -> (-57.448, 66.4157)
  line L376 (-56.2748, 65.2837) -> (-55.3673, 62.8959)
  line L377 (-55.3673, 62.8959) -> (-54.4874, 65.2837)
  line L378 (-54.4874, 65.2837) -> (-56.2748, 65.2837)
  spline S587 degree 2 poles (-61.9898, 66.5394) (-61.9898, 66.8923) (-61.6827, 66.8923) knots 0 0 0 1 1 1
  spline S588 degree 2 poles (-61.6827, 66.8923) (-61.4811, 66.8923) (-61.3482, 66.6998) knots 0 0 0 1 1 1
  line L379 (-61.3482, 66.6998) -> (-59.0017, 63.1067)
  line L380 (-59.0017, 63.1067) -> (-59.0017, 66.5302)
  spline S589 degree 2 poles (-59.0017, 66.5302) (-59.0017, 66.8923) (-58.6533, 66.8923) knots 0 0 0 1 1 1
  spline S590 degree 2 poles (-58.6533, 66.8923) (-58.305, 66.8923) (-58.305, 66.5302) knots 0 0 0 1 1 1
  line L381 (-58.305, 66.5302) -> (-58.305, 62.2039)
  spline S591 degree 2 poles (-58.305, 62.2039) (-58.305, 61.8601) (-58.635, 61.8601) knots 0 0 0 1 1 1
  spline S592 degree 2 poles (-58.635, 61.8601) (-58.855, 61.8601) (-59.0154, 62.0985) knots 0 0 0 1 1 1
  line L382 (-59.0154, 62.0985) -> (-61.2932, 65.5999)
  line L383 (-61.2932, 65.5999) -> (-61.2932, 62.2222)
  spline S593 degree 2 poles (-61.2932, 62.2222) (-61.2932, 61.8601) (-61.6415, 61.8601) knots 0 0 0 1 1 1
  spline S594 degree 2 poles (-61.6415, 61.8601) (-61.9898, 61.8601) (-61.9898, 62.2222) knots 0 0 0 1 1 1
  line L384 (-61.9898, 62.2222) -> (-61.9898, 66.5394)
  spline S595 degree 2 poles (-66.4399, 66.379) (-66.4811, 66.4615) (-66.4811, 66.5486) knots 0 0 0 1 1 1
  spline S596 degree 2 poles (-66.4811, 66.5486) (-66.4811, 66.6861) (-66.2612, 66.8923) (-66.1191, 66.8923) knots 0 0 0 1 2 2 2
  spline S597 degree 2 poles (-66.1191, 66.8923) (-65.9403, 66.8923) (-65.8258, 66.6998) knots 0 0 0 1 1 1
  line L385 (-65.8258, 66.6998) -> (-64.318, 64.0096)
  line L386 (-64.318, 64.0096) -> (-63.7772, 64.5825)
  line L387 (-63.7772, 64.5825) -> (-63.7772, 66.5302)
  spline S598 degree 2 poles (-63.7772, 66.5302) (-63.7772, 66.8923) (-63.4289, 66.8923) knots 0 0 0 1 1 1
  spline S599 degree 2 poles (-63.4289, 66.8923) (-63.076, 66.8923) (-63.076, 66.5302) knots 0 0 0 1 1 1
  line L388 (-63.076, 66.5302) -> (-63.076, 62.2405)
  spline S600 degree 2 poles (-63.076, 62.2405) (-63.076, 61.8785) (-63.4289, 61.8785) knots 0 0 0 1 1 1
  spline S601 degree 2 poles (-63.4289, 61.8785) (-63.7772, 61.8785) (-63.7772, 62.2405) knots 0 0 0 1 1 1
  line L389 (-63.7772, 62.2405) -> (-63.7772, 63.7438)
  line L390 (-63.7772, 63.7438) -> (-65.5462, 61.9793)
  spline S602 degree 2 poles (-65.5462, 61.9793) (-65.647, 61.8785) (-65.7662, 61.8785) knots 0 0 0 1 1 1
  spline S603 degree 2 poles (-65.7662, 61.8785) (-65.9128, 61.8785) (-66.1191, 62.103) (-66.1191, 62.236) knots 0 0 0 1 2 2 2
  spline S604 degree 2 poles (-66.1191, 62.236) (-66.1191, 62.378) (-66.0228, 62.4789) knots 0 0 0 1 1 1
  line L391 (-66.0228, 62.4789) -> (-64.8267, 63.5834)
  line L392 (-64.8267, 63.5834) -> (-66.4399, 66.379)
  line L393 (-72.077, 62.268) -> (-71.2383, 66.5807)
  spline S605 degree 2 poles (-71.2383, 66.5807) (-71.1742, 66.9015) (-70.8396, 66.9015) knots 0 0 0 1 1 1
  spline S606 degree 2 poles (-70.8396, 66.9015) (-70.5005, 66.9015) (-70.4134, 66.5898) knots 0 0 0 1 1 1
  line L394 (-70.4134, 66.5898) -> (-69.5793, 63.2626)
  line L395 (-69.5793, 63.2626) -> (-68.8002, 66.6127)
  spline S607 degree 2 poles (-68.8002, 66.6127) (-68.7268, 66.9015) (-68.3877, 66.9015) knots 0 0 0 1 1 1
  spline S608 degree 2 poles (-68.3877, 66.9015) (-68.044, 66.9015) (-67.9844, 66.6082) knots 0 0 0 1 1 1
  line L396 (-67.9844, 66.6082) -> (-67.0953, 62.323)
  spline S609 degree 2 poles (-67.0953, 62.323) (-67.0586, 62.1214) (-67.2694, 61.8785) (-67.4344, 61.8785) knots 0 0 0 1 2 2 2
  spline S610 degree 2 poles (-67.4344, 61.8785) (-67.714, 61.8785) (-67.7644, 62.126) knots 0 0 0 1 1 1
  line L397 (-67.7644, 62.126) -> (-68.4243, 65.6136)
  line L398 (-68.4243, 65.6136) -> (-69.2264, 62.1489)
  spline S611 degree 2 poles (-69.2264, 62.1489) (-69.2905, 61.8785) (-69.5747, 61.8785) knots 0 0 0 1 1 1
  spline S612 degree 2 poles (-69.5747, 61.8785) (-69.8451, 61.8785) (-69.9047, 62.0985) knots 0 0 0 1 1 1
  line L399 (-69.9047, 62.0985) -> (-70.7663, 65.577)
  line L400 (-70.7663, 65.577) -> (-71.385, 62.1626)
  spline S613 degree 2 poles (-71.385, 62.1626) (-71.44, 61.8785) (-71.7195, 61.8785) knots 0 0 0 1 1 1
  spline S614 degree 2 poles (-71.7195, 61.8785) (-71.8845, 61.8785) (-72.0999, 62.1168) (-72.077, 62.268) knots 0 0 0 1 2 2 2
  spline S615 degree 2 poles (-77.0358, 66.4157) (-77.0588, 66.4844) (-77.0588, 66.5486) knots 0 0 0 1 1 1
  spline S616 degree 2 poles (-77.0588, 66.5486) (-77.0588, 66.6998) (-76.8296, 66.8923) (-76.6921, 66.8923) knots 0 0 0 1 2 2 2
  spline S617 degree 2 poles (-76.6921, 66.8923) (-76.4584, 66.8923) (-76.3805, 66.6723) knots 0 0 0 1 1 1
  line L401 (-76.3805, 66.6723) -> (-76.0963, 65.9803)
  line L402 (-76.0963, 65.9803) -> (-73.8598, 65.9803)
  line L403 (-73.8598, 65.9803) -> (-73.5986, 66.6677)
  spline S618 degree 2 poles (-73.5986, 66.6677) (-73.5023, 66.8923) (-73.2686, 66.8923) knots 0 0 0 1 1 1
  spline S619 degree 2 poles (-73.2686, 66.8923) (-72.9157, 66.8923) (-72.9157, 66.5532) knots 0 0 0 1 1 1
  spline S620 degree 2 poles (-72.9157, 66.5532) (-72.9157, 66.489) (-72.934, 66.434) knots 0 0 0 1 1 1
  line L404 (-72.934, 66.434) -> (-74.5931, 62.0572)
  spline S621 degree 2 poles (-74.5931, 62.0572) (-74.7352, 61.8418) (-74.946, 61.8418) knots 0 0 0 1 1 1
  spline S622 degree 2 poles (-74.946, 61.8418) (-75.1568, 61.8418) (-75.3035, 62.0526) knots 0 0 0 1 1 1
  line L405 (-75.3035, 62.0526) -> (-77.0358, 66.4157)
  line L406 (-75.8626, 65.2837) -> (-74.9551, 62.8959)
  line L407 (-74.9551, 62.8959) -> (-74.0752, 65.2837)
  line L408 (-74.0752, 65.2837) -> (-75.8626, 65.2837)
  line L409 (-14.5509, 70.3018) -> (-12.9835, 70.3018)
  line L410 (-12.9835, 70.3018) -> (-12.9835, 75.4256)
  spline S623 degree 2 poles (-12.9835, 75.4256) (-12.9835, 75.7877) (-12.6169, 75.7877) knots 0 0 0 1 1 1
  spline S624 degree 2 poles (-12.6169, 75.7877) (-12.2548, 75.7877) (-12.2548, 75.4256) knots 0 0 0 1 1 1
  line L411 (-12.2548, 75.4256) -> (-12.2548, 70.3018)
  line L412 (-12.2548, 70.3018) -> (-10.6829, 70.3018)
  spline S625 degree 2 poles (-10.6829, 70.3018) (-10.3208, 70.3018) (-10.3208, 69.9306) knots 0 0 0 1 1 1
  spline S626 degree 2 poles (-10.3208, 69.9306) (-10.3208, 69.5685) (-10.6829, 69.5685) knots 0 0 0 1 1 1
  line L413 (-10.6829, 69.5685) -> (-14.5509, 69.5685)
  spline S627 degree 2 poles (-14.5509, 69.5685) (-14.9176, 69.5685) (-14.9176, 69.9306) knots 0 0 0 1 1 1
  spline S628 degree 2 poles (-14.9176, 69.9306) (-14.9176, 70.3018) (-14.5509, 70.3018) knots 0 0 0 1 1 1
  spline S629 degree 2 poles (-19.5235, 72.0525) (-19.5235, 72.8087) (-19.0515, 73.157) knots 0 0 0 1 1 1
  spline S630 degree 2 poles (-19.0515, 73.157) (-18.6757, 73.4641) (-18.3319, 73.4641) knots 0 0 0 1 1 1
  line L414 (-18.3319, 73.4641) -> (-18.2907, 73.4595)
  line L415 (-18.2907, 73.4595) -> (-19.4548, 75.0773)
  spline S631 degree 2 poles (-19.4548, 75.0773) (-19.5235, 75.1873) (-19.5235, 75.2881) knots 0 0 0 1 1 1
  spline S632 degree 2 poles (-19.5235, 75.2881) (-19.5235, 75.4348) (-19.3081, 75.6502) (-19.166, 75.6502) knots 0 0 0 1 2 2 2
  spline S633 degree 2 poles (-19.166, 75.6502) (-19.0011, 75.6502) (-18.9598, 75.5402) knots 0 0 0 1 1 1
  line L416 (-18.9598, 75.5402) -> (-17.5116, 73.4641)
  line L417 (-17.5116, 73.4641) -> (-16.6637, 73.4641)
  line L418 (-16.6637, 73.4641) -> (-16.6637, 75.2881)
  spline S634 degree 2 poles (-16.6637, 75.2881) (-16.6637, 75.6502) (-16.3154, 75.6502) knots 0 0 0 1 1 1
  spline S635 degree 2 poles (-16.3154, 75.6502) (-15.9671, 75.6502) (-15.9671, 75.2881) knots 0 0 0 1 1 1
  line L419 (-15.9671, 75.2881) -> (-15.9671, 70.6364)
  line L420 (-15.9671, 70.6364) -> (-18.0753, 70.6364)
  spline S636 degree 2 poles (-18.0753, 70.6364) (-18.6757, 70.6364) (-19.079, 70.9938) knots 0 0 0 1 1 1
  spline S637 degree 2 poles (-19.079, 70.9938) (-19.5235, 71.3926) (-19.5235, 72.0525) knots 0 0 0 1 1 1
  spline S638 degree 2 poles (-18.8269, 72.0525) (-18.8269, 71.7088) (-18.3915, 71.3421) (-18.0753, 71.3421) knots 0 0 0 1 2 2 2
  line L421 (-18.0753, 71.3421) -> (-16.6637, 71.3421)
  line L422 (-16.6637, 71.3421) -> (-16.6637, 72.7583)
  line L423 (-16.6637, 72.7583) -> (-18.3319, 72.7583)
  spline S639 degree 2 poles (-18.3319, 72.7583) (-18.4603, 72.7583) (-18.6207, 72.6116) knots 0 0 0 1 1 1
  spline S640 degree 2 poles (-18.6207, 72.6116) (-18.8269, 72.4192) (-18.8269, 72.0525) knots 0 0 0 1 1 1
  spline S641 degree 2 poles (-21.2742, 75.279) (-21.2742, 75.641) (-20.9168, 75.641) knots 0 0 0 1 1 1
  spline S642 degree 2 poles (-20.9168, 75.641) (-20.5639, 75.641) (-20.5639, 75.279) knots 0 0 0 1 1 1
  line L424 (-20.5639, 75.279) -> (-20.5639, 70.9893)
  spline S643 degree 2 poles (-20.5639, 70.9893) (-20.5639, 70.6272) (-20.9168, 70.6272) knots 0 0 0 1 1 1
  spline S644 degree 2 poles (-20.9168, 70.6272) (-21.2742, 70.6272) (-21.2742, 70.9893) knots 0 0 0 1 1 1
  line L425 (-21.2742, 70.9893) -> (-21.2742, 75.279)
  spline S645 degree 2 poles (-25.8114, 74.2294) (-25.8114, 75.6685) (-24.0103, 75.6685) knots 0 0 0 1 1 1
  spline S646 degree 2 poles (-24.0103, 75.6685) (-22.9608, 75.6685) (-22.3696, 74.6007) knots 0 0 0 1 1 1
  spline S647 degree 2 poles (-22.3696, 74.6007) (-22.3237, 74.5228) (-22.3237, 74.4265) knots 0 0 0 1 1 1
  spline S648 degree 2 poles (-22.3237, 74.4265) (-22.3237, 74.2707) (-22.5529, 74.0415) (-22.7041, 74.0415) knots 0 0 0 1 2 2 2
  spline S649 degree 2 poles (-22.7041, 74.0415) (-22.8829, 74.0415) (-22.9654, 74.2203) knots 0 0 0 1 1 1
  spline S650 degree 2 poles (-22.9654, 74.2203) (-23.3045, 74.9719) (-24.0103, 74.9719) knots 0 0 0 1 1 1
  spline S651 degree 2 poles (-24.0103, 74.9719) (-25.1102, 74.9719) (-25.1102, 74.2432) knots 0 0 0 1 1 1
  spline S652 degree 2 poles (-25.1102, 74.2432) (-25.1102, 73.8536) (-24.4915, 73.5695) knots 0 0 0 1 1 1
  spline S653 degree 2 poles (-24.4915, 73.5695) (-23.7536, 73.2716) (-23.1304, 73.0195) knots 0 0 0 1 1 1
  spline S654 degree 2 poles (-23.1304, 73.0195) (-22.3742, 72.5887) (-22.3742, 71.8738) knots 0 0 0 1 1 1
  spline S655 degree 2 poles (-22.3742, 71.8738) (-22.3742, 70.6043) (-23.9278, 70.5401) knots 0 0 0 1 1 1
  spline S656 degree 2 poles (-23.9278, 70.5401) (-24.5236, 70.5126) (-25.4448, 71.0626) (-25.6235, 71.6034) knots 0 0 0 1 2 2 2
  spline S657 degree 2 poles (-25.6235, 71.6034) (-25.651, 71.663) (-25.651, 71.718) knots 0 0 0 1 1 1
  spline S658 degree 2 poles (-25.651, 71.718) (-25.651, 72.0388) (-25.289, 72.0388) knots 0 0 0 1 1 1
  spline S659 degree 2 poles (-25.289, 72.0388) (-25.0369, 72.0388) (-24.959, 71.8004) knots 0 0 0 1 1 1
  spline S660 degree 2 poles (-24.959, 71.8004) (-24.8673, 71.5301) (-24.3036, 71.2184) (-23.9599, 71.2367) knots 0 0 0 1 2 2 2
  spline S661 degree 2 poles (-23.9599, 71.2367) (-23.0845, 71.278) (-23.0845, 71.8554) knots 0 0 0 1 1 1
  spline S662 degree 2 poles (-23.0845, 71.8554) (-23.0845, 72.2633) (-23.6941, 72.5337) knots 0 0 0 1 1 1
  spline S663 degree 2 poles (-23.6941, 72.5337) (-24.4457, 72.85) (-25.0552, 73.0791) knots 0 0 0 1 1 1
  spline S664 degree 2 poles (-25.0552, 73.0791) (-25.8114, 73.5007) (-25.8114, 74.2294) knots 0 0 0 1 1 1
  line L426 (-30.0324, 71.3605) -> (-28.85, 71.3605)
  line L427 (-28.85, 71.3605) -> (-28.85, 75.2881)
  spline S665 degree 2 poles (-28.85, 75.2881) (-28.85, 75.6594) (-28.4925, 75.6594) knots 0 0 0 1 1 1
  spline S666 degree 2 poles (-28.4925, 75.6594) (-28.1304, 75.6594) (-28.1304, 75.2881) knots 0 0 0 1 1 1
  line L428 (-28.1304, 75.2881) -> (-28.1304, 71.3605)
  line L429 (-28.1304, 71.3605) -> (-26.9526, 71.3605)
  spline S667 degree 2 poles (-26.9526, 71.3605) (-26.5905, 71.3605) (-26.5905, 70.9984) knots 0 0 0 1 1 1
  spline S668 degree 2 poles (-26.5905, 70.9984) (-26.5905, 70.6364) (-26.9526, 70.6364) knots 0 0 0 1 1 1
  line L430 (-26.9526, 70.6364) -> (-30.0324, 70.6364)
  spline S669 degree 2 poles (-30.0324, 70.6364) (-30.399, 70.6364) (-30.399, 70.9984) knots 0 0 0 1 1 1
  spline S670 degree 2 poles (-30.399, 70.9984) (-30.399, 71.3605) (-30.0324, 71.3605) knots 0 0 0 1 1 1
  spline S671 degree 2 poles (-35.2799, 75.1644) (-35.3029, 75.2331) (-35.3029, 75.2973) knots 0 0 0 1 1 1
  spline S672 degree 2 poles (-35.3029, 75.2973) (-35.3029, 75.4485) (-35.0737, 75.641) (-34.9362, 75.641) knots 0 0 0 1 2 2 2
  spline S673 degree 2 poles (-34.9362, 75.641) (-34.7025, 75.641) (-34.6246, 75.421) knots 0 0 0 1 1 1
  line L431 (-34.6246, 75.421) -> (-34.3404, 74.729)
  line L432 (-34.3404, 74.729) -> (-32.1039, 74.729)
  line L433 (-32.1039, 74.729) -> (-31.8427, 75.4165)
  spline S674 degree 2 poles (-31.8427, 75.4165) (-31.7464, 75.641) (-31.5127, 75.641) knots 0 0 0 1 1 1
  spline S675 degree 2 poles (-31.5127, 75.641) (-31.1598, 75.641) (-31.1598, 75.3019) knots 0 0 0 1 1 1